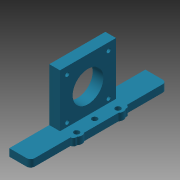
# Autodesk Inventor part: StepperMotorPlate
Saved by Autodesk Inventor 2014 SP1 (Build 180222100, 222)
## iProperties
Created: 2015-11-01
Part Number: StepperMotorPlate
Material: PPS Plastic
Document SubType Name: Modeling
Designer: Daniel Sikar
Density: 1.637 g/cm^3
Appearance: Turquoise
Mass: 12.9619 g
Surface Area: 51.1729 cm^2
Volume: 7.9181 cm^3
Author: Daniel Sikar
Autodesk Inventor part; units mm, degrees
ref_plane "YZ Plane" through (0, 0, 0) normal (1, 0, 0) x (0, 1, 0)
ref_plane "XZ Plane" through (0, 0, 0) normal (0, 1, 0) x (-1, 0, 0)
ref_plane "XY Plane" through (0, 0, 0) normal (0, 0, 1) x (1, 0, 0)
sketch "Sketch1" plane through (0, 0, 0) normal (0, 0, 1) x (1, 0, 0)
  circle A0 centre (0, 0) radius 11.5
  circle A1 centre (-15.5, 15.5) radius 1.5
  circle A2 centre (-15.5, -15.5) radius 1.5
  circle A3 centre (15.5, 15.5) radius 1.5
  circle A4 centre (15.5, -15.5) radius 1.5
  line L0 (-21, -24) -> (21, -24)
  line L1 (0, 20) -> (4.5462, 20) construction
  line L2 (-21, 21) -> (-1, 21)
  line L3 (1, 21) -> (21, 21)
  line L4 (-21, 21) -> (-21, 5.9161)
  line L5 (-21, -5.9161) -> (-21, -24)
  line L6 (21, 21) -> (21, 5.9161)
  line L7 (21, -5.9161) -> (21, -24)
  line L8 (-1.865, 21) -> (1.6498, 21)
  line L9 (-21, 8.451) -> (-21, -8.8551)
  line L10 (21, 10.9387) -> (21, -8.8551)
  dimension "d0" = 23
  dimension "d1" = 3
  dimension "d2" = 3
  dimension "d3" = 24
  dimension "d5" = 8.5
  constraints: 22 end point, 6 perpendicular, 6 point on line, 5 centre point, 4 parallel, 2 horizontal, 1 coincident
  measures "d0" diameter of A0
  measures "d1" diameter of A1
  measures "d2" diameter of A2
  measures "d3" distance from line of L0 point (0, 0)
  measures "d5" distance from line of L0 A2.centre
extrude "Extrusion1" add sketch "Sketch1" along normal blind 4
sketch "Sketch2" plane through (0, 0, 4) normal (0, 0, 1) x (1, 0, 0)
  line L0 (-21, -24) -> (21, -24) projected
  line L1 (21, -24) -> (21, 21) projected
  line L2 (-21, -24) -> (21, -24)
  line L3 (21, -24) -> (21, -18.5)
  line L4 (21, -18.5) -> (-21, -18.5)
  line L5 (-21, -18.5) -> (-21, -24)
  dimension "d9" = 5.5
  constraints: 8 end point, 2 parallel, 1 horizontal, 1 perpendicular, 1 point on line
  measures "d9" distance of L3.end L2.end
extrude "Extrusion2" add sketch "Sketch2" along normal blind 10
sketch "Sketch3" plane through (-21, -24, 0) normal (0, -1, 0) x (1, 0, 0)
  line L0 (42, 0) -> (42, 14) projected
  line L1 (0, 0) -> (0, 14) projected
  circle A0 centre (5.5, 11) radius 2
  circle A1 centre (36.5, 11) radius 2
  line L2 (0, 4) -> (42, 4) projected
  circle A2 centre (21, 9) radius 2
  line L3 (0, 14) -> (42, 14) projected
  point P0 (21, 0)
  dimension "d12" = 4
  dimension "d13" = 4
  dimension "d16" = 5.5
  dimension "d17" = 5.5
  dimension "d18" = 7
  dimension "d19" = 7
  dimension "d27" = 4
  dimension "d28" = 5
  constraints: 3 centre point
  measures "d12" diameter of A1
  measures "d13" diameter of A0
  measures "d16" distance from line of A0.centre L1
  measures "d17" distance from line of L0 A1.centre
  measures "d18" distance from line of L2 A1.centre
  measures "d19" distance from line of A0.centre L2
  measures "d27" diameter of A2
  measures "d28" distance from line of L3 A2.centre
sketch "Sketch4" plane through (-21, -24, 0) normal (0, -1, 0) x (1, 0, 0)
  circle A0 centre (5.5, 11) radius 2 projected
  circle A1 centre (36.5, 11) radius 2 projected
  arc A2 (8.1458, 14) -> (2.8542, 14) centre (5.5, 11) ccw
  arc A3 (39.1458, 14) -> (33.8542, 14) centre (36.5, 11) ccw
  line L0 (42, 14) -> (0, 14) projected
  line L1 (2.8542, 14) -> (8.1458, 14)
  line L2 (33.8542, 14) -> (39.1458, 14)
  point P0 (21, 0)
  dimension "d22" = 8
  dimension "d23" = 8
  constraints: 4 end point, 4 point on circle, 2 centre point, 2 coincident
  measures "d22" diameter of A2
  measures "d23" diameter of A3
extrude "Extrusion4" add sketch "Sketch4" against normal blind 5.5 contours L0 A2 | A3 L0
fillet "Fillet1" radius 2 2 edges at (-21, -21.25, 14) (21, -21.25, 14)
extrude "Extrusion5" cut sketch "Sketch3" against normal blind 5.5 contours A0 | A1 | A2
sketch "Sketch5" plane through (0, 0, 0) normal (0, 0, -1) x (-1, 0, 0)
  circle A0 centre (0, 0) radius 11.5 projected
  circle A1 centre (-15.5, -15.5) radius 1.5 projected
  circle A2 centre (-15.5, 15.5) radius 1.5 projected
  circle A3 centre (15.5, -15.5) radius 1.5 projected
  circle A4 centre (15.5, 15.5) radius 1.5 projected
  line L0 (-21, -24) -> (21, -24) projected
  line L1 (21, -24) -> (21, 21) projected
  line L2 (21, 21) -> (-21, 21) projected
  line L3 (-21, 21) -> (-21, -24) projected
extrude "Extrusion6" add sketch "Sketch5" along normal blind 4
sketch "Sketch6" plane through (-21, -18.5, 4) normal (-1, 0, 0) x (0, 0, 1)
  line L0 (-8, -5.5) -> (-8, 39.5) projected
  line L1 (8, -5.5) -> (-8, -5.5) projected
  line L2 (8, -5.5) -> (-8, -5.5)
  line L3 (-8, -5.5) -> (-8, 0)
  line L4 (-8, 0) -> (8, 0)
  line L5 (8, 0) -> (8, -5.5)
  point P0 (-4, 18.5)
  constraints: 8 end point, 2 parallel, 1 horizontal, 1 perpendicular, 1 point on line
extrude "Extrusion7" add sketch "Sketch6" along normal blind 30
sketch "Sketch7" plane through (21, -18.5, 4) normal (1, 0, 0) x (0, 0, -1)
  line L0 (-8, -5.5) -> (-8, 0) projected
  line L1 (8, -5.5) -> (-8, -5.5) projected
  line L2 (-8, 0) -> (8, 0)
  line L3 (8, 0) -> (8, -5.5)
  line L4 (8, -5.5) -> (-8, -5.5)
  line L5 (-8, -5.5) -> (-8, 0)
  point P0 (4, 18.5)
  constraints: 8 end point, 2 parallel, 1 horizontal, 1 perpendicular
extrude "Extrusion8" add sketch "Sketch7" along normal blind 30
fillet "Fillet2" radius 3 2 edges at (51, -21.25, 12) (-51, -21.25, 12)
body "Solid1"
